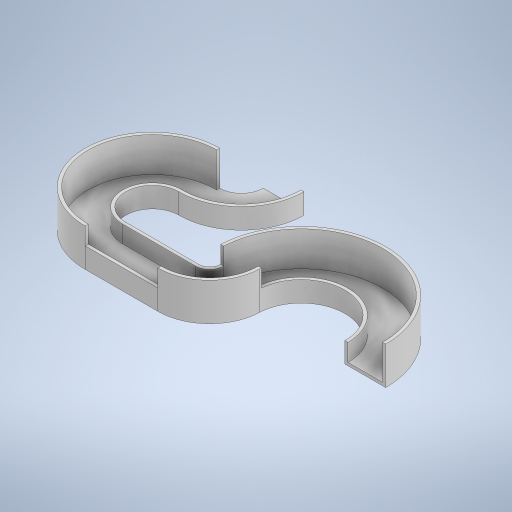
# Autodesk Inventor part: Agrupar bolinhas novamente
Saved by Autodesk Inventor 2024 (Build 280153000, 153)
## iProperties
Created: 2023-05-19
Part Number: Agrupar bolinhas novamente
Material: Genérico
Document SubType Name: Modeling
Designer: jpjoa
Density: 1 g/cm^3
Appearance: Padrão
Author: jpjoa
Autodesk Inventor part; units mm, degrees
ref_plane "YZ Plane" through (0, 0, 0) normal (1, 0, 0) x (0, 1, 0)
ref_plane "XZ Plane" through (0, 0, 0) normal (0, 1, 0) x (-1, 0, 0)
ref_plane "XY Plane" through (0, 0, 0) normal (0, 0, 1) x (1, 0, 0)
sketch "Esboço1" plane through (0, 0, 0) normal (0, 1, 0) x (-1, 0, 0)
  arc A0 (24.3813, -38.6705) -> (73.0565, -39.6571) centre (48.7289, -38.6705) ccw
  arc A1 (98.3571, -15.3618) -> (73.0565, -39.6571) centre (98.3571, -40.6831) ccw
  line L0 (98.3571, -15.3618) -> (136.2408, -15.3618)
  arc A2 (136.2408, -82.1618) -> (136.2408, -15.3618) centre (136.2408, -48.7618) ccw
  arc A3 (136.2408, -82.1618) -> (123.3076, -95.095) centre (136.2408, -95.095) ccw
  arc A4 (136.2408, -64.1618) -> (105.3076, -95.095) centre (136.2408, -95.095) ccw
  arc A5 (136.2408, -64.1618) -> (136.2408, -33.3618) centre (136.2408, -48.7618) ccw
  line L1 (136.2408, -33.3618) -> (98.3571, -33.3618)
  arc A6 (98.3571, -33.3618) -> (91.0417, -40.3865) centre (98.3571, -40.6831) ccw
  arc A7 (6.3813, -38.6705) -> (91.0417, -40.3865) centre (48.7289, -38.6705) ccw
  arc A8 (4.7813, -38.6705) -> (92.6404, -40.4513) centre (48.7289, -38.6705) ccw
  arc A9 (98.3571, -34.9618) -> (92.6404, -40.4513) centre (98.3571, -40.6831) ccw
  line L2 (98.3571, -34.9618) -> (136.2408, -34.9618)
  arc A10 (136.2408, -62.5618) -> (136.2408, -34.9618) centre (136.2408, -48.7618) ccw
  arc A11 (136.2408, -62.5618) -> (103.7076, -95.095) centre (136.2408, -95.095) ccw
  arc A12 (25.9813, -38.6705) -> (71.4578, -39.5923) centre (48.7289, -38.6705) ccw
  arc A13 (98.3571, -13.7618) -> (71.4578, -39.5923) centre (98.3571, -40.6831) ccw
  line L3 (98.3571, -13.7618) -> (136.2408, -13.7618)
  arc A14 (136.2408, -83.7618) -> (136.2408, -13.7618) centre (136.2408, -48.7618) ccw
  arc A15 (136.2408, -83.7618) -> (124.9076, -95.095) centre (136.2408, -95.095) ccw
  line L4 (25.9813, -38.6705) -> (4.7813, -38.6705)
  line L5 (124.9076, -95.095) -> (103.7076, -95.095)
  line L6 (92.6304, -40.6831) -> (91.0286, -40.6831)
  line L7 (71.3873, -40.6831) -> (72.9932, -40.6831)
  line L8 (136.2408, -15.3618) -> (136.2408, -13.7618)
  line L9 (136.2408, -83.7618) -> (136.2408, -82.1618)
  line L10 (98.3571, -15.3618) -> (98.3571, -13.7618)
  point P0 (0, 0)
  point P1 (117.2989, -33.3618)
  point P2 (136.2408, -82.9618)
  point P3 (136.2408, -14.5618)
  point P4 (91.8295, -40.6831)
  point P5 (72.1902, -40.6831)
  point P6 (24.3813, -38.6705)
  point P7 (6.3813, -38.6705)
  point P8 (136.2408, -83.7618)
  dimension "d10" = 18
  dimension "d11" = 30.8
  dimension "d12" = 1.6
  dimension "d13" = 1.6
  constraints: 38 point on circle, 22 end point, 16 centre point, 10 horizontal alignment, 6 vertical alignment, 5 horizontal, 5 midpoint, 3 tangent, 2 vertical, 12 other
  measures "d10" radial gap between concentric circles of A3 A4
  measures "d11" distance of L1.start A4.start
  measures "d12" radial gap between concentric circles of A7 A8
  measures "d13" radial gap between concentric circles of A1 A13
extrude "Extrusão1" add sketch "Esboço1" against normal blind 1.6
extrude "Extrusão2" add sketch "Esboço1" along normal blind 18 contours L7 A12 A13 L10 A1 A0 | A7 L6 A8 L4 | L8 A14 L9 A2
extrude "Extrusão3" add sketch "Esboço1" along normal blind 9 contours L4 A12 L7 A0 | A7 A6 L1 A5 A4 L5 A11 A10 L2 A9 A8 L6 | L10 L3 L8 L0
equation "\"d10\" = Esfera"
equation "\"d12\" = Margem"
equation "\"d13\" = Margem"
equation "\"Esfera\" = 18"
equation "\"Margem\" = 1.6"
